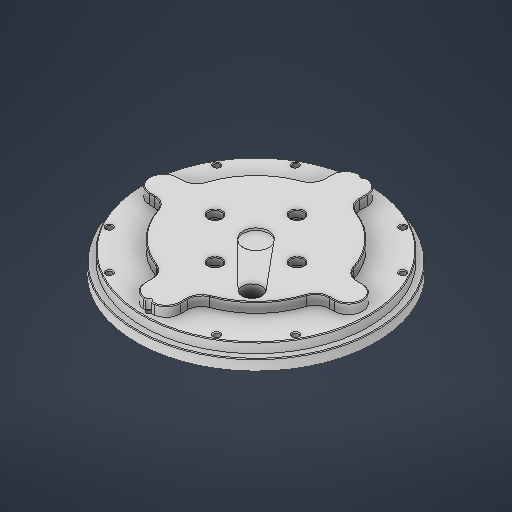
# Autodesk Inventor part: Build Plateform one Indents
Saved by Autodesk Inventor 2025 (Build 290162000, 162)
## iProperties
Created: 2024-08-23
Part Number: Build Plateform one Indents
Material: Generic
Document SubType Name: Modeling
Designer: mayhe
Density: 1 g/cm^3
Appearance: Default
Author: mayhe
Autodesk Inventor part; units mm, degrees
ref_plane "YZ Plane" through (0, 0, 0) normal (1, 0, 0) x (0, 1, 0)
ref_plane "XZ Plane" through (0, 0, 0) normal (0, 1, 0) x (-1, 0, 0)
ref_plane "XY Plane" through (0, 0, 0) normal (0, 0, 1) x (1, 0, 0)
sketch "Sketch1" plane through (0, 0, 0) normal (0, 1, 0) x (-1, 0, 0)
  circle A0 centre (0, 0) radius 84.5
  circle A1 centre (0, 0) radius 80
  circle A2 centre (0, 0) radius 76
  line L0 (65, 0) -> (65, 0)
  line L1 (-2.5, -76) -> (2.5, -76)
  line L2 (2.5, 76) -> (-2.5, 76)
  line L3 (-12.5, -76) -> (12.5, 76) construction
  line L4 (12.5, -76) -> (-12.5, 76) construction
  line L5 (-75.339233, 0) -> (-75.339233, 0)
  line L6 (75.339233, 0) -> (75.339233, 0)
  line L7 (75.339233, 10) -> (-75.339233, -10) construction
  line L8 (-75.339233, 10) -> (75.339233, -10) construction
  arc A3 (65.339233, -10) -> (75.339233, 0) centre (65.339233, 0) ccw
  arc A4 (75.339233, 0) -> (65.339233, 10) centre (65.339233, 0) ccw
  arc A5 (12.5, 66) -> (2.5, 76) centre (2.5, 66) ccw
  arc A6 (-2.5, 76) -> (-12.5, 66) centre (-2.5, 66) ccw
  arc A7 (2.5, -76) -> (12.5, -66) centre (2.5, -66) ccw
  arc A8 (-12.5, -66) -> (-2.5, -76) centre (-2.5, -66) ccw
  arc A9 (-75.339233, 0) -> (-65.339233, -10) centre (-65.339233, 0) ccw
  arc A10 (-65.339233, 10) -> (-75.339233, 0) centre (-65.339233, 0) ccw
  arc A11 (-52.331725, -16.923077) -> (-19.038462, -51.599777) centre (0, 0) ccw
  arc A12 (19.038462, -51.599777) -> (52.331725, -16.923077) centre (0, 0) ccw
  arc A13 (52.331725, 16.923077) -> (19.038462, 51.599777) centre (0, 0) ccw
  arc A14 (-19.038462, 51.599777) -> (-52.331725, 16.923077) centre (0, 0) ccw
  line L9 (12.5, -66) -> (12.5, -60.981555)
  line L10 (12.5, -1.659162) -> (12.5, 1.659162)
  line L11 (12.5, 60.981555) -> (12.5, 66)
  line L12 (-12.5, 66) -> (-12.5, 60.981555)
  line L13 (-12.5, -60.981555) -> (-12.5, -66)
  line L14 (-65.339233, -10) -> (-61.846584, -10)
  line L15 (61.846584, -10) -> (65.339233, -10)
  line L16 (65.339233, 10) -> (61.846584, 10)
  line L17 (-61.846584, 10) -> (-65.339233, 10)
  arc A15 (-12.5, -60.981555) -> (-19.038462, -51.599777) centre (-22.5, -60.981555) ccw
  arc A16 (-52.331725, -16.923077) -> (-61.846584, -10) centre (-61.846584, -20) ccw
  arc A17 (-61.846584, 10) -> (-52.331725, 16.923077) centre (-61.846584, 20) ccw
  arc A18 (-19.038462, 51.599777) -> (-12.5, 60.981555) centre (-22.5, 60.981555) ccw
  arc A19 (12.5, 60.981555) -> (19.038462, 51.599777) centre (22.5, 60.981555) ccw
  arc A20 (52.331725, 16.923077) -> (61.846584, 10) centre (61.846584, 20) ccw
  arc A21 (61.846584, -10) -> (52.331725, -16.923077) centre (61.846584, -20) ccw
  arc A22 (19.038462, -51.599777) -> (12.5, -60.981555) centre (22.5, -60.981555) ccw
  point P0 (-54.083269, 10)
  point P1 (-54.083269, -10)
  point P2 (-12.5, -53.560713)
  point P3 (12.5, -53.560713)
  point P4 (54.083269, -10)
  point P5 (54.083269, 10)
  point P6 (12.5, 53.560713)
  point P7 (-12.5, 53.560713)
  point P8 (3.918132, 75.898934)
  point P9 (-3.918132, 75.898934)
  point P10 (-3.918132, -75.898934)
  point P11 (3.918132, -75.898934)
  point P12 (75.339233, 0)
  point P13 (0, -76)
  point P14 (0, 76)
  dimension "d26" = 152
  dimension "d24" = 169
  dimension "d25" = 160
  dimension "d27" = 25
  dimension "d29" = 20
  dimension "d30" = 10
  dimension "d31" = 10
  dimension "d32" = 10
  constraints: 48 point on circle, 42 tangent, 36 end point, 22 centre point, 18 point on line, 13 equal radius, 12 parallel, 5 perpendicular, 4 midpoint, 3 coincident, 3 horizontal, 3 other
  measures "d24" diameter of A0
  measures "d25" diameter of A1
  measures "d27" distance of L4.end L3.end
  measures "d29" distance of L7.end L8.start
  measures "d30" radius of A3
  measures "d31" radius of A15
  measures "d32" radius of A18
extrude "Extrusion1" add sketch "Sketch1" along normal blind 21.5 contours A5 L11 A19 A13 A20 L16 A4 A3 L15 A21 A12 A22 L9 A7 A2 A8 L13 A15 A11 A16 L14 A9 A10 L17 A17 A14 A18 L12 A6
extrude "Extrusion2" add sketch "Sketch1" along normal blind 14.5 contours A1 | A2 A7 L9 A22 A12 A21 L15 A3 A4 L16 A20 A13 A19 L11 A5 | A2 L2 A5 | A7 L1 A2 | A2 A6 L2 | L1 A8 A2 | A6 L12 A18 A14 A17 L17 A10 A9 L14 A16 A11 A15 L13 A8 A2
extrude "Extrusion3" add sketch "Sketch1" along normal blind 7.5 contours A0
sketch "Sketch2" plane through (0, 21.5, 0) normal (0, 1, 0) x (1, 0, 0)
  circle A0 centre (0, 0) radius 29
  circle A1 centre (0, 29) radius 4.5
  circle A2 centre (0, 29) radius 2.5
  circle A3 centre (-29, 0) radius 4.5
  circle A4 centre (-29, 0) radius 2.5
  circle A5 centre (0, -29) radius 4.5
  circle A6 centre (0, -29) radius 2.5
  circle A7 centre (29, 0) radius 4.5
  circle A8 centre (29, 0) radius 2.5
  dimension "d40" = 58
  dimension "d41" = 9
  dimension "d42" = 5
  dimension "d45" = 360
  constraints: 8 centre point, 5 coincident, 1 vertical alignment, 19 other
  measures "d41" diameter of A1
  measures "d42" diameter of A2
extrude "Extrusion4" cut sketch "Sketch2" against normal blind 5 contours A0 A8 | A0 A8 | A8 A0 A7 | A0 A7 A8 | A1 A0 A2 | A0 A2 A1 | A5 A0 A6 | A0 A6 A5 | A2 A0 | A0 A2 | A6 A0 | A0 A6 | A3 A0 A4 | A0 A4 A3 | A4 A0 | A0 A4
hole "Hole1" at (29, 21.5, 0) at (0, 21.5, 29) at (-29, 21.5, 0) at (0, 21.5, -29) direction (0, -1, 0) diameter 5.5 end through all
sketch "Sketch3" plane through (0, 21.5, 0) normal (0, 1, 0) x (1, 0, 0)
  circle A0 centre (0, 0) radius 76
  circle A1 centre (0, 76) radius 1.75
  circle A2 centre (0, -76) radius 1.75
  dimension "d56" = 152
  dimension "d57" = 3.5
  dimension "d60" = 360
  constraints: 2 centre point, 1 coincident, 1 vertical alignment, 7 other
  measures "d57" diameter of A1
hole "Hole2" at (0, 21.5, -76) at (0, 21.5, 76) direction (0, -1, 0) diameter 3.242 depth 21.5 counterbore diameter 4 counterbore depth 7 thread size "M4x0.7" class "6H" standard "ANSI Metric M Profile"
sketch "Sketch4" plane through (0, 0, 0) normal (0, -1, 0) x (1, 0, 0)
  arc A0 (-20.845089, 35.305556) -> (20.845089, 35.305556) centre (0, 0) ccw
  line L0 (18.303005, 36) -> (-18.303005, 36)
  circle A1 centre (0, 0) radius 10
  arc A2 (20.845089, 35.305556) -> (18.303005, 36) centre (18.303005, 31) ccw
  arc A3 (-18.303005, 36) -> (-20.845089, 35.305556) centre (-18.303005, 31) ccw
  point P0 (19.621417, 36)
  point P1 (-19.621417, 36)
  dimension "d69" = 82
  dimension "d70" = 5
  dimension "d71" = 20
  dimension "d162" = 5
  constraints: 8 point on circle, 4 centre point, 4 tangent, 2 coincident, 2 end point, 2 point on line, 1 equal radius, 1 horizontal
  measures "d69" diameter of A0
  measures "d70" distance edge to line of A0 L0
  measures "d71" diameter of A1
  measures "d162" radius of A2
extrude "Extrusion5" cut sketch "Sketch4" against normal blind 1.5
extrude "Extrusion6" cut sketch "Sketch4" against normal blind 12 contours A1
sketch "Sketch5" plane through (0, 14.5, 0) normal (0, 1, 0) x (1, 0, 0)
  circle A0 centre (0, 0) radius 10
  arc A1 (-1.620908, 75.982713) -> (1.620908, 75.982713) centre (0, 76) ccw
  circle A2 centre (0, 0) radius 76
  arc A3 (1.620908, -75.982713) -> (-1.620908, -75.982713) centre (0, -76) ccw
  circle A4 centre (0, -76) radius 2.5
  circle A5 centre (38, -65.817931) radius 2.5
  circle A6 centre (65.817931, -38) radius 2.5
  circle A7 centre (76, 0) radius 2.5
  circle A8 centre (65.817931, 38) radius 2.5
  circle A9 centre (38, 65.817931) radius 2.5
  circle A10 centre (0, 76) radius 2.5
  circle A11 centre (-38, 65.817931) radius 2.5
  circle A12 centre (-65.817931, 38) radius 2.5
  circle A13 centre (-76, 0) radius 2.5
  circle A14 centre (-65.817931, -38) radius 2.5
  circle A15 centre (-38, -65.817931) radius 2.5
  dimension "d76" = 5
  dimension "d79" = 360
  constraints: 13 centre point, 2 coincident, 1 point on circle, 25 other
  measures "d76" diameter of A4
hole "Hole3" at (-38, 14.5, 65.817931) at (-65.817931, 14.5, 38) at (-65.817931, 14.5, -38) at (-38, 14.5, -65.817931) at (38, 14.5, -65.817931) at (65.817931, 14.5, -38) at (65.817931, 14.5, 38) at (38, 14.5, 65.817931) direction (0, -1, 0) diameter 4.134 end through all thread size "M5x0.8" class "6H" standard "ANSI Metric M Profile"
chamfer "Chamfer1" distance 0.5 angle 45 30 edges at (39.6742, 21.5, 38.0914) (55.9631, 21.5, 11.9139) (63.5929, 21.5, 10) (75.3392, 21.5, 0) (63.5929, 21.5, -10) (55.9631, 21.5, -11.9139) (39.6742, 21.5, -38.0914) (14.2959, 21.5, -55.2638) (12.5, 21.5, -63.4908) (10.0558, 21.5, -72.5505) (14.2959, 21.5, 55.2638) (12.5, 21.5, 63.4908) (10.0558, 21.5, 72.5505) (-14.2959, 21.5, 55.2638) (-12.5, 21.5, 63.4908) (-10.0558, 21.5, 72.5505) (-39.6742, 21.5, 38.0914) (-55.9631, 21.5, 11.9139) (-63.5929, 21.5, 10) (-75.3392, 21.5, 0) (-63.5929, 21.5, -10) (-55.9631, 21.5, -11.9139) (-39.6742, 21.5, -38.0914) (-14.2959, 21.5, -55.2638) (-12.5, 21.5, -63.4908) (-10.0558, 21.5, -72.5505) (-4.5, 21.5, 29) (-33.5, 21.5, 0) (-4.5, 21.5, -29) (24.5, 21.5, 0)
chamfer "Chamfer2" distance 0.5 angle 45 2 edges at (80, 14.5, 0) (84.5, 7.5, 0)
sketch "Sketch7" plane through (0, 21.5, 0) normal (0, 1, 0) x (1, 0, 0)
  circle A0 centre (0, 0) radius 47.5
  circle A1 centre (47.5, 0) radius 2.5
  circle A2 centre (43.884278, 18.177463) radius 2.5
  circle A3 centre (33.587572, 33.587572) radius 2.5
  circle A4 centre (18.177463, 43.884278) radius 2.5
  circle A5 centre (0, 47.5) radius 2.5
  circle A6 centre (-18.177463, 43.884278) radius 2.5
  circle A7 centre (-33.587572, 33.587572) radius 2.5
  circle A8 centre (-43.884278, 18.177463) radius 2.5
  circle A9 centre (-47.5, 0) radius 2.5
  circle A10 centre (-43.884278, -18.177463) radius 2.5
  circle A11 centre (-33.587572, -33.587572) radius 2.5
  circle A12 centre (-18.177463, -43.884278) radius 2.5
  circle A13 centre (0, -47.5) radius 2.5
  circle A14 centre (18.177463, -43.884278) radius 2.5
  circle A15 centre (33.587572, -33.587572) radius 2.5
  circle A16 centre (43.884278, -18.177463) radius 2.5
  dimension "d107" = 95
  dimension "d108" = 5
  dimension "d111" = 360
  constraints: 16 centre point, 1 coincident, 1 horizontal alignment, 35 other
  measures "d108" diameter of A1
hole "Hole5" [suppressed]
sketch "Sketch9" plane through (0, 21.5, 0) normal (0, 1, 0) x (1, 0, 0)
  circle A0 centre (0, 0) radius 9.125
  circle A1 centre (0, 0) radius 40
  circle A2 centre (-40, 0) radius 9.125
  circle A3 centre (-28.284271, -28.284271) radius 9.125
  circle A4 centre (0, -40) radius 9.125
  circle A5 centre (28.284271, -28.284271) radius 9.125
  circle A6 centre (40, 0) radius 9.125
  circle A7 centre (28.284271, 28.284271) radius 9.125
  circle A8 centre (0, 40) radius 9.125
  circle A9 centre (-28.284271, 28.284271) radius 9.125
  dimension "d140" = 80
  dimension "d139" = 18.25
  dimension "d141" = 18.25
  dimension "d144" = 360
  constraints: 9 centre point, 2 coincident, 1 horizontal alignment, 19 other
  measures "d139" diameter of A0
  measures "d141" diameter of A2
extrude "Extrusion9" cut sketch "Sketch9" against normal blind 1.5 contours A0
sketch "Sketch10" plane through (0, 21.5, 0) normal (0, 1, 0) x (1, 0, 0)
  circle A0 centre (30.382264, -33.195151) radius 7
  circle A1 centre (0, 45) radius 7
  point P0 (0, 0)
  dimension "d151" = 14
  dimension "d152" = 45
  dimension "d158" = 14
  dimension "d159" = 45
  constraints: 2 centre point
  measures "d151" diameter of A0
  measures "d152" distance of point (0, 0) A0.centre
  measures "d158" diameter of A1
  measures "d159" distance of A1.centre point (0, 0)
extrude "Extrusion10" cut sketch "Sketch10" against normal through all contours A0
chamfer "Chamfer4" distance 0.5 angle 45 8 edges at (-38, 14.5, 63.7509) (-65.8179, 14.5, 35.933) (-65.8179, 14.5, -40.067) (-38, 14.5, -67.8849) (38, 14.5, -67.8849) (65.8179, 14.5, -40.067) (65.8179, 14.5, 35.933) (38, 14.5, 63.7509)
sketch "Sketch11" plane through (0, 21.5, 0) normal (0, 1, 0) x (1, 0, 0)
  circle A0 centre (30.382264, -33.195151) radius 7
  line L0 (25.447513, -38.159849) -> (-6.432801, -6.471839)
  circle A1 centre (0, 0) radius 9.125
  line L1 (35.763372, -28.718134) -> (7.014659, 5.836111)
  point P0 (9.082812, -0.876445)
  point P1 (-6.432801, -6.471839)
  point P2 (32.104534, -26.41033)
  constraints: 4 end point, 4 point on circle, 4 tangent
extrude "Extrusion11" cut sketch "Sketch11" against normal blind 1
body "Solid1"
